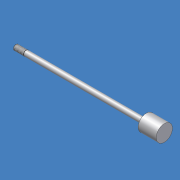
# Autodesk Inventor part: 044-DXP0_rod
Saved by Autodesk Inventor 2012 (Build 160160000, 160)
## iProperties
Category: PARTsolutions
Created: 2013-01-20
Part Number: 044-DXP0_rod
Catalog Web Link: www.cadenas.de
Description: Standard Air Cylinder_rod - Original Line - Standard Air Cylinders
Document SubType Name: Modeling
Designer: PARTsolutions
Material: Default
Density: 1 g/cm^3
NB: 044-DXP0_rod
NN: Standard Air Cylinder_rod
NT: Original Line - Standard Air Cylinders
NBSYN: $PN.$COLOR1._rod
LINA: 044-DXP0_rod
PN: 044-DXP
DASH: -
BORE: 0.75000000
BOREPN: 04
STROKE: 4.000
STROKEALG: [0.001:50/0.001]
STROKE1: 4.000
ACTING: D
ACTINGALG: '' , 'Single Acting' , 'R' , 'Reverse Single Acting' , 'D' , 'Double Acting'
ACTINGPN: D
MNT: XP
MNTALG: '' , 'Front Nose Mounting' , 'P' , 'Rear Pivot Mounting' , 'XP' , 'Double End or Pivot Mounting' , 'X' , 'Double End Mounting' , 'BF' , 'Front Block Mounting' , 'BR' , 'Rear Block Mounting for Vertical Positioning' , 'BFT' , 'Front Block Trunnion Mounting' , 'BRT' , 'Rear Block Trunnion Mounting'
MNTPN: XP
DERALG: '' , 'N/A'
NRALG: '' , 'N/A'
BMALG: '' , 'N/A'
COALG: '' , 'N/A'
MALG: '', 'Without Magnet', 'M', 'With Magnet'
EEL: 0
EEMAX: 46
EEALG: '', 'Without Extra Extension', 'EE', 'With Extra Extension'
EELALG: 0
EEPN1: 0.000
KALG: '', 'Standard' , 'K' , 'Ports Rotated 90deg'
QALG: '' , 'Without Side Ported Rear Head' , 'Q' , 'With Side Ported Rear Head'
YALG: '' , 'Without Pivot Bushing' , 'Y' , 'With Pivot Bushing'
FALG: '', 'Standard', 'F', 'Molycoated Body'
TALG: '' , 'Standard' , 'N' , 'Low Temperature' , 'V' , 'High Temperature'
BALG: '', 'Without Bumper' , 'B' , 'With Bumper'
HALG: '', 'N/A'
SERALG: '' , 'Without Spring Extend/Return' , 'JS' , 'With Spring Return' , 'JR' , 'With Spring Extend'
SRALG: 'C' , 'Carbon Steel Rod' , 'SR' , '303 Stainless Steel Rod' , '' , '303 Stainless Steel Rod1'
SRCON: 0
WALG: '' , 'Without Wiper' , 'W' , 'With Wiper'
EALG: '' , 'Without Special Lube and Seals' , 'E' , 'With Special Lube and Seals'
HLALG: '' , 'Wihout Low Pressure Hydraulic' , 'HL' , 'With Low Pressure Hydraulic'
STALG: '' , 'Without Switch Track' , 'T' , 'With Switch Track'
STPALG: '' , 'N/A'
PRCALG: '' , 'Without Piston Rod Clevis' , 'D-166-1' , 'With Piston Rod Clevis'
PBALG: '' , 'Without Pivot Bracket' , 'D-167' , 'With Pivot Bracket'
TLEN: 5.2555
TEXT: 0.367
SPACE: 0.210
FRAC: 22.7500
RGDACCON: R
RHCON: P
RHCONON: 1
FNUTCON: 1
RNUTCON: 1
FNUTPN: D-9
RNUTPN: D-9
FNUTTRANS: 0.0000
RNUTTRANS: 0.0000
VHOLECON: 0
A1: 1.5940
A1N: 0.8750
A1P: 1.5940
A1B: 1.5940
A4: 0.2525
A4N: 0.3130
A4P: 0.2525
A5: 0.0300
A1H: 1.594
A1NH: 0.5310
A1PH: 1.5940
A1BH: 1.0940
A1SH: 1.2190
A2H: 0.2190
A2NH: 0.2190
LENGTH: 3.7500
LENGTH1: 3.7500
LENGTH2: 3.8100
MUL: 4.0000
MUL11: 4.0000
MUL22: 10.7600
MUL33: 6.7600
MUL2: 4.0000
MUL211: 4.0000
MUL222: 2.6900
MUL233: 1.6900
SSS: 8.0000
RGLEN: 1.3715
RHLEN: 1.1230
SSS1: 5.0000
A13: 1.3120
THDLEN1: 0.5000
THD1: 0.2500
TAB: UNF
THDLEN: 0.5000
THD: 0.2500
OD: 0.7615
RODL: 6.9380
PL: 0.8440
RODDIA: 0.2500
HEX: 0.2500
RODTRANS: 0.0000
G1: 0.1250
ON: 0
G5: 0.6250
DERLEN: 6.0940
THOLE: 0.0000
WF: 0.2200
BADD: 0.0000
MADD: 0.0000
NVADD: 0.000
JRADD: 0.00000
COLOR: 0.71,0.71,0.71,0.00
GROOVE: 1
HOL: 1
D7: 0.2520
H1: 1.1175
D1: 0.8625
D1RH: 0.8625
D1P: 0.8325
D1B: 0.8625
D1N: 0.8050
D1NRH: 0.8050
D1BRH: 0.8325
D1PRH: 0.8625
BOZO: 0
HADD: 0.000
COLOR1: 0
DEFL: 0.0000
HEXL: 0.0000
SSADD: 0.0000
WFL: 0.0000
MOVE: 0.0000
KT: DUMMY
SUPPLIER: Bimba
ARTICLENO: 044-DXP0_rod
BOMINFO: 044-DXP0_rod
CREATOR: CADENAS GmbH
PSOL_IDENT_0: {\\10.0.0.242\data_v9\23d-libs\bimba\bimba\bimba_imperial\bimba_full_line\original_line_cylinders\st
PSOL_IDENT_1: andard_air_cylinders\rod.prj},278 {VTYP=3D},{NB=044-DXP0_rod},{LINA=044-DXP0_rod},{NN=Standard Air C
PSOL_IDENT_2: ylinder_rod},{DATE=11.09.2012 07:37:40},{GEOMDATE=06.09.2012 09:06:00},{VERSION=},{LINEID=50},{LINES
PSOL_IDENT_3: UBID=-1},{WBVAR=STROKE,ACTING,MNT,DER,NR,BM,CO,M,EE,EEL,K,Q,Y,F,G,T,B,H,SER,SR,NT,W,E,HL,ST,STP,PRC,
PSOL_IDENT_4: PB,COLOR1}  {NB=044-DXP0_rod},{LINA=044-DXP0_rod},{KT=DUMMY},{PN=044-DXP},{DASH=-},{BORE=0.75000000}
PSOL_IDENT_5: ,{BOREPN=04},{STROKE=4.000},{STROKEALG=[0.001:50/0.001]},{STROKE1=4.000},{ACTING=D},{ACTINGALG= '' ,
PSOL_IDENT_6: 'Single Acting' , 'R' , 'Reverse Single Acting' , 'D' , 'Double Acting' },{ACTINGPN=D},{MNT=XP},{MN
PSOL_IDENT_7: TALG= '' , 'Front Nose Mounting' , 'P' , 'Rear Pivot Mounting' , 'XP' , 'Double End or Pivot Mountin
PSOL_IDENT_8: g' , 'X' , 'Double End Mounting' , 'BF' , 'Front Block Mounting' , 'BR' , 'Rear Block Mounting for V
PSOL_IDENT_9: ertical Positioning' , 'BFT' , 'Front Block Trunnion Mounting' , 'BRT' , 'Rear Block Trunnion Mounti
PSOL_IDENT_10: ng' },{TYPE=},{MNTPN=XP},{DER=},{DERALG= '' , 'N/A' },{NR=},{NRALG= '' , 'N/A' },{NRPN=},{BM=},{BMAL
PSOL_IDENT_11: G= '' , 'N/A' },{BMPN=},{CO=},{COALG= '' , 'N/A' },{M=},{MALG= '', 'Without Magnet', 'M', 'With Magn
PSOL_IDENT_12: et' },{EE=},{EEL=0},{EEMAX=46},{EEALG= '', 'Without Extra Extension', 'EE', 'With Extra Extension' }
PSOL_IDENT_13: ,{EELALG=0},{EEPN=},{EEPN1=0.000},{K=},{KALG= '', 'Standard' , 'K' , 'Ports Rotated 90deg' },{KPN=},
PSOL_IDENT_14: {Q=},{QALG= '' , 'Without Side Ported Rear Head' , 'Q' , 'With Side Ported Rear Head' },{QPN=},{Y=},
PSOL_IDENT_15: {YALG= '' , 'Without Pivot Bushing' , 'Y' , 'With Pivot Bushing' },{YPN=},{F=},{FALG= '', 'Standard'
PSOL_IDENT_16: , 'F', 'Molycoated Body' },{FPN=},{G=},{GPN=},{T=},{TALG= '' , 'Standard' , 'N' , 'Low Temperature'
PSOL_IDENT_17: , 'V' , 'High Temperature' },{NPN=},{VPN=},{B=},{BALG= '', 'Without Bumper' , 'B' , 'With Bumper' },
PSOL_IDENT_18: {BPN=},{H=},{HALG= '', 'N/A' },{HPN=},{SER=},{SERALG= '' , 'Without Spring Extend/Return' , 'JS' , '
PSOL_IDENT_19: With Spring Return' , 'JR' , 'With Spring Extend' },{SR=},{SRALG= 'C' , 'Carbon Steel Rod' , 'SR' ,
PSOL_IDENT_20: '303 Stainless Steel Rod' , '' , '303 Stainless Steel Rod1' },{SRPN=},{SRCON=0},{NT=},{NTPN=},{W=},{
PSOL_IDENT_21: WALG= '' , 'Without Wiper' , 'W' , 'With Wiper' },{WPN=},{E=},{EALG= '' , 'Without Special Lube and
PSOL_IDENT_22: Seals' , 'E' , 'With Special Lube and Seals' },{EPN=},{HL=},{HLALG= '' , 'Wihout Low Pressure Hydrau
PSOL_IDENT_23: lic' , 'HL' , 'With Low Pressure Hydraulic' },{ST=},{STALG= '' , 'Without Switch Track' , 'T' , 'Wit
PSOL_IDENT_24: h Switch Track' },{STP=},{STPALG= '' , 'N/A' },{STPN=},{PRC=},{PRCALG= '' , 'Without Piston Rod Clev
PSOL_IDENT_25: is' , 'D-166-1' , 'With Piston Rod Clevis' },{PRCPN=},{PB=},{PBALG= '' , 'Without Pivot Bracket' , '
PSOL_IDENT_26: D-167' , 'With Pivot Bracket' },{PBPN=},{TLEN=5.2555},{TEXT=0.366667},{SPACE=0.209524},{FRAC=22.7500
PSOL_IDENT_27: },{RGCON=},{RGDACCON=R},{RHCON=P},{RHCONON=1},{RHACCON=},{FNUTCON=1},{RNUTCON=1},{FNUTPN=D-9},{RNUTP
PSOL_IDENT_28: N=D-9},{FNUTTRANS=0.0000},{RNUTTRANS=0.0000},{VHOLECON=0},{A1=1.5940},{A1N=0.8750},{A1P=1.5940},{A1B
PSOL_IDENT_29: =1.5940},{A4=0.2525},{A4N=0.3130},{A4P=0.2525},{A5=0.0300},{A1H=1.594},{A1NH=0.5310},{A1PH=1.5940},{
PSOL_IDENT_30: A1BH=1.0940},{A1SH=1.2190},{A2H=0.2190},{A2NH=0.2190},{LENGTH=3.7500},{LENGTH1=3.7500},{LENGTH2=3.81
PSOL_IDENT_31: 00},{MUL=4.0000},{MUL11=4.0000},{MUL22=10.7600},{MUL33=6.7600},{MUL2=4.0000},{MUL211=4.0000},{MUL222
PSOL_IDENT_32: =2.6900},{MUL233=1.6900},{SSS=8.0000},{RGLEN=1.3715},{RHLEN=1.1230},{SSS1=5.0000},{A13=1.3120},{THDL
PSOL_IDENT_33: EN1=0.5000},{THD1=0.2500},{TAB=UNF},{THDLEN=0.5000},{THD=0.2500},{OD=0.7615},{RODL=6.9380},{PL=0.844
PSOL_IDENT_34: 0},{RODDIA=0.2500},{HEX=0.2500},{RODTRANS=0.0000},{G1=0.1250},{ON=0},{G5=0.6250},{DERLEN=6.0940},{TH
PSOL_IDENT_35: OLE=0.0000},{WF=0.2200},{BADD=0.0000},{MADD=0.0000},{NVADD=0.000},{JRADD=0.00000},{COLOR=0.71,0.71,0
PSOL_IDENT_36: .71,0.00},{GROOVE=1},{HOL=1},{D7=0.2520},{H1=1.1175},{D1=0.8625},{D1RH=0.8625},{D1P=0.8325},{D1B=0.8
PSOL_IDENT_37: 625},{D1N=0.8050},{D1NRH=0.8050},{D1BRH=0.8325},{D1PRH=0.8625},{BOZO=0},{HADD=0.000},{COLOR1=0},{DEF
PSOL_IDENT_38: L=0.0000},{HEXL=0.0000},{SSADD=0.0000},{WFL=0.0000},{MOVE=0.0000}
Title: 044-DXP0_rod
Author: Cadenas PARTsolutions
Comments: Original Line - Standard Air Cylinders
Autodesk Inventor part; units mm, degrees
sketch "Sketch_1" plane through (0, 0, 0) normal (0, 0, 1) x (1, 0, 0)
  line L0 (163.5252, 0) -> (0, 0)
  line L1 (0, 0) -> (0, 3.175)
  line L2 (0, 3.175) -> (142.0876, 3.175)
  line L3 (142.0876, 3.175) -> (142.0876, 9.6203)
  line L4 (142.0876, 9.6203) -> (163.5252, 9.6203)
  line L5 (163.5252, 9.6203) -> (163.5252, 0)
  line L6 (163.5252, 0) -> (0, 0)
  constraints: 14 end point
revolve "Revolution1" add sketch "Sketch_1" angle 360 about axis through (163.5252, 0, 0) along (1, 0, 0)
sketch "Sketch_3" plane through (0, 0, 0) normal (0, 0, 1) x (1, 0, 0)
  line L0 (0, 0) -> (-12.7, 0)
  line L1 (-12.7, 0) -> (-12.7, 2.634)
  line L2 (-12.7, 2.634) -> (-12.159, 3.175)
  line L3 (-12.159, 3.175) -> (0, 3.175)
  line L4 (0, 3.175) -> (0, 0)
  line L5 (0, 0) -> (-12.7, 0)
  constraints: 12 end point
revolve "Revolution2" add sketch "Sketch_3" angle 360 about axis through (0, 0, 0) along (1, 0, 0)
thread "Thread1" size "1/4-28 UNF" class "3A" standard "ANSI Unified Screw Threads" length 12.7 offset 142.0876
sketch "Sketch_30" plane through (0, 0, 0) normal (0, 0, 1) x (1, 0, 0)
  line L0 (0, 0) -> (-0.254, 0)
  line L1 (-0.254, 3.429) -> (-0.254, 2.921)
  line L2 (-0.254, 2.921) -> (0, 2.921)
  line L3 (0, 2.921) -> (0, 3.429)
  line L4 (0, 3.429) -> (-0.254, 3.429)
  constraints: 10 end point
revolve "Revolution3" cut sketch "Sketch_30" angle 360 about axis through (0, 0, 0) along (1, 0, 0)
ref_plane "rod_cp_XY" through (0, 0, 0) normal (1, 0, 0) x (0, 0, -1)
ref_plane "rod_cp_YZ" through (0, 0, 0) normal (0, 0, -1) x (0, 1, 0)
ref_plane "rod_cp_ZX" through (0, 0, 0) normal (0, 1, 0) x (1, 0, 0)
ref_plane "to_rod_clevis_XY" through (-12.7, 0, 0) normal (1, 0, 0) x (0, 0, -1)
ref_plane "to_rod_clevis_YZ" through (-12.7, 0, 0) normal (0, 0, -1) x (0, 1, 0)
ref_plane "to_rod_clevis_ZX" through (-12.7, 0, 0) normal (0, 1, 0) x (1, 0, 0)
ref_plane "rl2_XY" through (0, 0, 0) normal (1, 0, 0) x (0, 0, -1)
ref_plane "rl2_YZ" through (0, 0, 0) normal (0, 0, -1) x (0, 1, 0)
ref_plane "rl2_ZX" through (0, 0, 0) normal (0, 1, 0) x (1, 0, 0)
ref_plane "rl1_XY" through (-12.7, 0, 0) normal (1, 0, 0) x (0, 0, -1)
ref_plane "rl1_YZ" through (-12.7, 0, 0) normal (0, 0, -1) x (0, 1, 0)
ref_plane "rl1_ZX" through (-12.7, 0, 0) normal (0, 1, 0) x (1, 0, 0)
ref_plane "thd1_XY" through (-12.7, 3.175, 0) normal (1, 0, 0) x (0, 0, -1)
ref_plane "thd1_YZ" through (-12.7, 3.175, 0) normal (0, 0, -1) x (0, 1, 0)
ref_plane "thd1_ZX" through (-12.7, 3.175, 0) normal (0, 1, 0) x (1, 0, 0)
ref_plane "thd2_XY" through (-12.7, -3.175, 0) normal (1, 0, 0) x (0, 0, -1)
ref_plane "thd2_YZ" through (-12.7, -3.175, 0) normal (0, 0, -1) x (0, 1, 0)
ref_plane "thd2_ZX" through (-12.7, -3.175, 0) normal (0, 1, 0) x (1, 0, 0)
ref_plane "dia1_XY" through (0, 3.175, 0) normal (1, 0, 0) x (0, 0, -1)
ref_plane "dia1_YZ" through (0, 3.175, 0) normal (0, 0, -1) x (0, 1, 0)
ref_plane "dia1_ZX" through (0, 3.175, 0) normal (0, 1, 0) x (1, 0, 0)
ref_plane "dia2_XY" through (0, -3.175, 0) normal (1, 0, 0) x (0, 0, -1)
ref_plane "dia2_YZ" through (0, -3.175, 0) normal (0, 0, -1) x (0, 1, 0)
ref_plane "dia2_ZX" through (0, -3.175, 0) normal (0, 1, 0) x (1, 0, 0)
ref_plane "hh1_XY" through (193.6496, 0, 0) normal (0, 0, 1) x (1, 0, 0)
ref_plane "hh1_YZ" through (193.6496, 0, 0) normal (1, 0, 0) x (0, 1, 0)
ref_plane "hh1_ZX" through (193.6496, 0, 0) normal (0, 1, 0) x (0, 0, 1)
ref_plane "hh2_XY" through (200.0504, 0, 0) normal (0, 0, 1) x (1, 0, 0)
ref_plane "hh2_YZ" through (200.0504, 0, 0) normal (1, 0, 0) x (0, 1, 0)
ref_plane "hh2_ZX" through (200.0504, 0, 0) normal (0, 1, 0) x (0, 0, 1)
ref_plane "dia12_XY" through (0, 0, 10.9537) normal (1, 0, 0) x (0, 0, -1)
ref_plane "dia12_YZ" through (0, 0, 10.9537) normal (0, 0, -1) x (0, 1, 0)
ref_plane "dia12_ZX" through (0, 0, 10.9537) normal (0, 1, 0) x (1, 0, 0)
ref_plane "dia22_XY" through (0, 0, -10.9537) normal (1, 0, 0) x (0, 0, -1)
ref_plane "dia22_YZ" through (0, 0, -10.9537) normal (0, 0, -1) x (0, 1, 0)
ref_plane "dia22_ZX" through (0, 0, -10.9537) normal (0, 1, 0) x (1, 0, 0)
body "Solid1"
